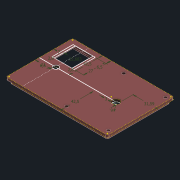
# Autodesk Inventor part: caja
Saved by Autodesk Inventor 2021 (Build 250183000, 183)
## iProperties
Created: 2021-12-14
Part Number: caja
Material: Generic
Document SubType Name: Modeling
Designer: Juan M. Casillas
Density: 1 g/cm^3
Appearance: Default
Author: Juan M. Casillas
Autodesk Inventor part; units mm, degrees
ref_plane "YZ Plane" through (0, 0, 0) normal (1, 0, 0) x (0, 1, 0)
ref_plane "XZ Plane" through (0, 0, 0) normal (0, 1, 0) x (-1, 0, 0)
ref_plane "XY Plane" through (0, 0, 0) normal (0, 0, 1) x (1, 0, 0)
sketch "Sketch1" plane through (0, 0, 0) normal (0, 1, 0) x (-1, 0, 0)
  line L0 (55, 45) -> (-55, 45)
  line L1 (-55, 45) -> (-55, -45)
  line L2 (-55, -45) -> (55, -45)
  line L3 (55, -45) -> (55, 45)
  line L4 (55, 45) -> (-55, -45) construction
  line L5 (-55, 45) -> (55, -45) construction
  line L6 (-12.1638, 34.5239) -> (-35.1638, 34.5239)
  line L7 (-35.1638, 34.5239) -> (-35.1638, 7.5239)
  line L8 (-35.1638, 7.5239) -> (-12.1638, 7.5239)
  line L9 (-12.1638, 7.5239) -> (-12.1638, 34.5239)
  line L10 (-12.1638, 34.5239) -> (-35.1638, 7.5239) construction
  line L11 (-35.1638, 34.5239) -> (-12.1638, 7.5239) construction
  circle A0 centre (-27.7205, -16.8019) radius 3.25
  line L12 (55, 0) -> (31, 0) construction
  circle A1 centre (31, 0) radius 4 construction
  circle A2 centre (31, 0) radius 40 construction
  point P0 (0, 0)
  point P1 (-23.6638, 21.0239)
  dimension "d1" = 110
  dimension "d2" = 90
  dimension "d3" = 23
  dimension "d4" = 27
  dimension "d5" = 6.5
  dimension "d6" = 24
  dimension "d7" = 8
  dimension "d8" = 80
  constraints: 26 end point, 5 midpoint, 4 parallel, 3 centre point, 3 horizontal, 2 coincident, 2 perpendicular
  measures "d1" distance of L2.end L1.end
  measures "d2" distance of L1.end L0.end
  measures "d3" distance of L8.end L7.end
  measures "d4" distance of L7.end L6.end
  measures "d5" diameter of A0
  measures "d6" distance of L12.start L12.end
  measures "d7" diameter of A1
  measures "d8" diameter of A2
sketch "Sketch2" plane through (0, 0, 0) normal (0, 1, 0) x (-1, 0, 0)
  line L0 (82.5, 45) -> (-40, 45)
  line L1 (-40, 45) -> (-40, -40)
  line L2 (-40, -40) -> (82.5, -40)
  line L3 (82.5, -40) -> (82.5, 45)
  line L4 (82.5, 45) -> (-40, -40) construction
  line L5 (-40, 45) -> (82.5, -40) construction
  point P0 (0, 0)
  dimension "d10" = 122.5
  dimension "d11" = 85
  constraints: 12 end point, 2 parallel, 1 horizontal, 1 perpendicular
  measures "d10" distance of L2.end L1.end
  measures "d11" distance of L1.end L0.end
extrude "Extrusion1" add sketch "Sketch2" along normal blind 3
sketch "Sketch3" plane through (0, 0, 0) normal (0, -1, 0) x (1, 0, 0)
  circle A0 centre (8.41, 2.5) radius 11.1
  circle A1 centre (8.41, 2.5) radius 14.1
  line L0 (40, 45) -> (40, -40) construction
  line L1 (-82.5, 45) -> (40, 45) construction
  line L2 (-82.5, -40) -> (-82.5, 45) construction
  line L3 (40, -40) -> (-82.5, -40) construction
  line L4 (40, 2.5) -> (-82.5, 2.5) construction
  circle A2 centre (8.41, 2.5) radius 4.5
  line L5 (-82.5, 2.5) -> (40, 2.5) construction
  dimension "d15" = 22.2
  dimension "d16" = 3
  dimension "d20" = 42.5
  dimension "d21" = 9
  dimension "d42" = 31.59
  constraints: 4 end point, 3 centre point, 2 coincident, 2 midpoint, 1 perpendicular, 1 point on line
  measures "d15" diameter of A0
  measures "d16" radial gap between concentric circles of A0 A1
  measures "d20" distance between parallel lines of L1 L4
  measures "d21" diameter of A2
  measures "d42" distance from line of L0 point (8.41, 2.5)
extrude "Extrusion2" add sketch "Sketch3" along normal blind 3.5 contours A1
thicken "Thicken1" operation add thickness 7 both sides no extend neighbours yes toward (-1, 0, 0) faces at (-82.5, 1, -11.6667)
fillet "Fillet1" radius 2 4 edges at (-89.5, 1.5, 45) (40, 1.5, 45) (40, 1.5, -40) (-89.5, 1.5, -40)
extrude "Extrusion3" cut sketch "Sketch3" against normal blind 10 contours A2
sketch "Sketch4" plane through (0, 0, 0) normal (0, -1, 0) x (1, 0, 0)
  arc A0 (-7.0479, 5.0014) -> (-5.1277, 6.4422) centre (-7.0479, 7.0014) ccw
  line L0 (-13.69, 5.0014) -> (-7.0479, 5.0014)
  arc A1 (-13.69, 5.0014) -> (-15.69, 3.0014) centre (-13.69, 3.0014) ccw
  line L1 (-15.69, 2.0014) -> (-15.69, 3.0014)
  arc A2 (-15.69, 2.0014) -> (-13.69, 0.0014) centre (-13.69, 2.0014) ccw
  line L2 (-7.0487, 0.0014) -> (-13.69, 0.0014)
  arc A3 (-5.1284, -1.4397) -> (-7.0487, 0.0014) centre (-7.0487, -1.9986) ccw
  arc A4 (-5.1277, 6.4422) -> (-5.1284, -1.4397) centre (8.41, 2.5) ccw
  circle A5 centre (8.41, 2.5) radius 14.1 projected
  line L3 (8.41, -14.9987) -> (8.41, 25.3428) construction
  arc A6 (21.9477, 6.4422) -> (23.8679, 5.0014) centre (23.8679, 7.0014) ccw
  line L4 (30.51, 5.0014) -> (23.8679, 5.0014)
  arc A7 (32.51, 3.0014) -> (30.51, 5.0014) centre (30.51, 3.0014) ccw
  arc A8 (21.9484, -1.4397) -> (21.9477, 6.4422) centre (8.41, 2.5) ccw
  arc A9 (23.8687, 0.0014) -> (21.9484, -1.4397) centre (23.8687, -1.9986) ccw
  line L5 (32.51, 2.0014) -> (32.51, 3.0014)
  arc A10 (30.51, 0.0014) -> (32.51, 2.0014) centre (30.51, 2.0014) ccw
  line L6 (23.8687, 0.0014) -> (30.51, 0.0014)
  point P0 (0, 0)
  point P1 (21.9477, 6.4422)
  point P2 (21.9484, -1.4397)
  constraints: 20 point on circle, 14 end point, 12 symmetric about line, 10 centre point, 1 concentric, 1 vertical, 5 other
extrude "Extrusion4" add sketch "Sketch4" along normal up to surface (3.5 mm away) contours A0 A4 A3 L2 A2 L1 A1 L0 | A6 L4 A7 L5 A10 L6 A9 A5
fillet "Fillet2" radius 2 16 edges at (27.189, 0, 5.0014) (31.9242, 0, 4.4156) (32.51, 0, 2.5014) (31.9242, 0, 0.5872) (27.1894, 0, 0.0014) (22.6683, 0, -0.3989) (8.41, 0, -11.6) (-5.8483, 0, -0.3989) (-10.3694, 0, 0.0014) (-15.1042, 0, 0.5872) (-15.69, 0, 2.5014) (-15.1042, 0, 4.4156) (-10.369, 0, 5.0014) (-5.8476, 0, 5.4017) (8.41, 0, 16.6) (22.6676, 0, 5.4017)
sketch "Sketch5" plane through (0, 0, 0) normal (0, -1, 0) x (1, 0, 0)
  arc A0 (-89.5, -38) -> (-87.5, -40) centre (-87.5, -38) ccw projected
  line L0 (38, -40) -> (-87.5, -40) projected
  arc A1 (38, -40) -> (40, -38) centre (38, -38) ccw projected
  line L1 (40, 43) -> (40, -38) projected
  arc A2 (40, 43) -> (38, 45) centre (38, 43) ccw projected
  line L2 (-87.5, 45) -> (38, 45) projected
  arc A3 (-87.5, 45) -> (-89.5, 43) centre (-87.5, 43) ccw projected
  line L3 (-89.5, -38) -> (-89.5, 43) projected
  line L4 (30.51, 7.0014) -> (23.8679, 7.0014) projected
  arc A4 (34.51, 3.0014) -> (30.51, 7.0014) centre (30.51, 3.0014) ccw projected
  line L5 (34.51, 2.0014) -> (34.51, 3.0014) projected
  arc A5 (30.51, -1.9986) -> (34.51, 2.0014) centre (30.51, 2.0014) ccw projected
  line L6 (23.8687, -1.9986) -> (30.51, -1.9986) projected
  arc A6 (-7.0487, -1.9986) -> (23.8687, -1.9986) centre (8.41, 2.5) ccw projected
  line L7 (-13.69, -1.9986) -> (-7.0487, -1.9986) projected
  arc A7 (-17.69, 2.0014) -> (-13.69, -1.9986) centre (-13.69, 2.0014) ccw projected
  line L8 (-17.69, 3.0014) -> (-17.69, 2.0014) projected
  arc A8 (-13.69, 7.0014) -> (-17.69, 3.0014) centre (-13.69, 3.0014) ccw projected
  line L9 (-7.0479, 7.0014) -> (-13.69, 7.0014) projected
  arc A9 (23.8679, 7.0014) -> (-7.0479, 7.0014) centre (8.41, 2.5) ccw projected
  line L10 (-84.9, 42.4) -> (35.4, 42.4)
  line L11 (37.4, 40.4) -> (37.4, -35.4)
  line L12 (35.4, -37.4) -> (-84.9, -37.4)
  line L13 (-86.9, -35.4) -> (-86.9, 40.4)
  arc A10 (-86.9, -35.4) -> (-84.9, -37.4) centre (-84.9, -35.4) ccw
  arc A11 (-84.9, 42.4) -> (-86.9, 40.4) centre (-84.9, 40.4) ccw
  arc A12 (37.4, 40.4) -> (35.4, 42.4) centre (35.4, 40.4) ccw
  arc A13 (35.4, -37.4) -> (37.4, -35.4) centre (35.4, -35.4) ccw
  line L14 (-84.9, -35.9) -> (35.4, -35.9)
  arc A14 (35.4, -35.9) -> (35.9, -35.4) centre (35.4, -35.4) ccw
  line L15 (35.9, -35.4) -> (35.9, 40.4)
  arc A15 (35.9, 40.4) -> (35.4, 40.9) centre (35.4, 40.4) ccw
  line L16 (35.4, 40.9) -> (-84.9, 40.9)
  arc A16 (-84.9, 40.9) -> (-85.4, 40.4) centre (-84.9, 40.4) ccw
  line L17 (-85.4, 40.4) -> (-85.4, -35.4)
  arc A17 (-85.4, -35.4) -> (-84.9, -35.9) centre (-84.9, -35.4) ccw
  point P0 (0, 0)
  dimension "d27" = 2.6
  dimension "d28" = 2
  dimension "d29" = 1.5
  constraints: 16 end point, 16 point on circle, 8 centre point, 8 tangent, 3 equal radius, 10 other
  measures "d27" distance between parallel lines of L3 L13
  measures "d28" radius of A10
  measures "d29" distance between parallel lines of L12 L14
extrude "Extrusion5" add sketch "Sketch5" along normal blind 4 contours L10 A12 L11 A13 L12 A10 L13 A11
fillet "Fillet3" radius 2 8 edges at (35.7536, 0, -35.7536) (35.9, 0, 2.5) (35.7536, 0, 40.7536) (-24.75, 0, 40.9) (-85.2536, 0, 40.7536) (-85.4, 0, 2.5) (-85.2536, 0, -35.7536) (-24.75, 0, -35.9)
sketch "Sketch6" plane through (0, -3.5, 0) normal (0, -1, 0) x (1, 0, 0)
  arc A0 (21.9477, 6.4422) -> (-5.1277, 6.4422) centre (8.41, 2.5) ccw construction
  arc A1 (-7.0479, 5.0014) -> (-5.1277, 6.4422) centre (-7.0479, 7.0014) ccw construction
  line L0 (-13.69, 5.0014) -> (-7.0479, 5.0014) construction
  arc A2 (-13.69, 5.0014) -> (-15.69, 3.0014) centre (-13.69, 3.0014) ccw construction
  line L1 (-15.69, 2.0014) -> (-15.69, 3.0014) construction
  arc A3 (-15.69, 2.0014) -> (-13.69, 0.0014) centre (-13.69, 2.0014) ccw construction
  line L2 (-7.0487, 0.0014) -> (-13.69, 0.0014) construction
  arc A4 (-5.1284, -1.4397) -> (-7.0487, 0.0014) centre (-7.0487, -1.9986) ccw construction
  arc A5 (-5.1284, -1.4397) -> (21.9484, -1.4397) centre (8.41, 2.5) ccw construction
  arc A6 (23.8687, 0.0014) -> (21.9484, -1.4397) centre (23.8687, -1.9986) ccw construction
  line L3 (30.51, 0.0014) -> (23.8687, 0.0014) construction
  arc A7 (30.51, 0.0014) -> (32.51, 2.0014) centre (30.51, 2.0014) ccw construction
  line L4 (32.51, 3.0014) -> (32.51, 2.0014) construction
  arc A8 (32.51, 3.0014) -> (30.51, 5.0014) centre (30.51, 3.0014) ccw construction
  line L5 (23.8679, 5.0014) -> (30.51, 5.0014) construction
  arc A9 (21.9477, 6.4422) -> (23.8679, 5.0014) centre (23.8679, 7.0014) ccw construction
  circle A10 centre (8.41, 2.5) radius 11.1 construction
  line L6 (-15.69, 2.5014) -> (32.51, 2.5014) construction
  line L7 (-15.69, 2.5014) -> (-10.69, 2.5014) construction
  point P0 (0, 0)
  point P1 (27.51, 2.5014)
  point P2 (27.51, 2.5014)
  dimension "d33" = 5
  dimension "d34" = 5
  constraints: 4 end point, 2 coincident, 2 midpoint, 2 point on line
  measures "d33" distance from line of L4 point (27.51, 2.501)
  measures "d34" distance of L6.start L7.end
hole "Hole1" at (-10.69, -3.5, 2.5014) at (27.51, -3.5, 2.5014) direction (0, 1, 0) diameter 3.42 depth 5
sketch "Sketch7" plane through (0, 3, 0) normal (0, 1, 0) x (1, 0, 0)
  circle A0 centre (8.41, -2.5) radius 4.5 construction
  arc A1 (-87.5, 40) -> (-89.5, 38) centre (-87.5, 38) ccw construction
  line L0 (-89.5, 38) -> (-89.5, -43) construction
  arc A2 (-89.5, -43) -> (-87.5, -45) centre (-87.5, -43) ccw construction
  line L1 (-87.5, -45) -> (38, -45) construction
  arc A3 (38, -45) -> (40, -43) centre (38, -43) ccw construction
  line L2 (40, -43) -> (40, 38) construction
  arc A4 (40, 38) -> (38, 40) centre (38, 38) ccw construction
  line L3 (38, 40) -> (-87.5, 40) construction
  line L4 (-68.5, 40) -> (-68.5, -45) construction
  line L5 (-40.8109, -2.5) -> (-89.5, -2.5) construction
  circle A5 centre (-68.5, -2.5) radius 3.3
  line L6 (-54.217, 33.5) -> (-82.5, 33.5)
  line L7 (-82.5, 33.5) -> (-82.5, 6.5)
  line L8 (-82.5, 6.5) -> (-54.217, 6.5)
  line L9 (-54.217, 6.5) -> (-54.217, 33.5)
  line L10 (-54.217, 33.5) -> (-57.017, 33.5)
  line L11 (-57.017, 33.5) -> (-57.017, 6.5)
  line L12 (-57.017, 6.5) -> (-54.217, 6.5)
  line L13 (-54.217, 6.5) -> (-54.217, 33.5)
  line L14 (-82.5, 33.5) -> (-79.7, 33.5)
  line L15 (-79.7, 33.5) -> (-79.7, 6.5)
  line L16 (-79.7, 6.5) -> (-82.5, 6.5)
  line L17 (-82.5, 6.5) -> (-82.5, 33.5)
  line L18 (8.41, -2.5) -> (-89.5, -2.5)
  point P0 (0, 0)
  dimension "d45" = 21
  dimension "d46" = 42.5
  dimension "d47" = 6.6
  dimension "d48" = 6.5
  dimension "d49" = 7
  dimension "d50" = 27
  dimension "d52" = 2.8
  dimension "d53" = 2.8
  dimension "d59" = 22.683
  constraints: 30 end point, 6 parallel, 5 perpendicular, 5 point on line, 3 horizontal, 3 midpoint, 1 centre point
  measures "d45" distance between parallel lines of L0 L4
  measures "d46" distance between parallel lines of L3 L5
  measures "d47" diameter of A5
  measures "d48" distance between parallel lines of L3 L6
  measures "d49" distance between parallel lines of L0 L7
  measures "d50" distance of L8.end L6.start
  measures "d52" distance of L12.end L11.end
  measures "d53" distance of L15.end L16.end
  measures "d59" distance between parallel lines of L11 L15
extrude "Extrusion6" cut sketch "Sketch7" against normal blind 4 contours L18 A5 | A5 L18 | L11 L8 L15 L6
sketch "Sketch8" plane through (0, 0, 0) normal (0, -1, 0) x (1, 0, 0)
  line L0 (-54.217, -6.5) -> (-54.217, -33.5) projected
  line L1 (-57.017, -6.5) -> (-54.217, -6.5) projected
  line L2 (-57.017, -33.5) -> (-57.017, -6.5) projected
  line L3 (-54.217, -33.5) -> (-57.017, -33.5) projected
  line L4 (-82.5, -33.5) -> (-79.7, -33.5) projected
  line L5 (-82.5, -6.5) -> (-82.5, -33.5) projected
  line L6 (-82.5, -6.5) -> (-54.217, -6.5) projected
  line L7 (-79.7, -6.5) -> (-79.7, -33.5) projected
  point P0 (0, 0)
extrude "Extrusion7" cut sketch "Sketch8" against normal blind 1.2
thicken "Thicken2" operation add thickness 0.2 both sides no extend neighbours yes toward (0, 0, 1) faces at (-72.139, 2.4, -6.5) (-57.017, 2.4, -15.5) (-64.578, 1.8, -33.5) (-79.7, 2.4, -24.5)
sketch "Sketch9" plane through (0, 3, 0) normal (0, 1, 0) x (1, 0, 0)
  circle A0 centre (8.41, -2.5) radius 40 construction
  line L0 (38, 38) -> (8.41, -2.5) construction
  line L1 (8.41, -2.5) -> (38, -43) construction
  line L2 (38, 38) -> (35.0503, 33.9628) construction
  line L3 (38, -43) -> (35.0503, -38.9628) construction
  line L4 (30.7963, -33.1402) -> (-23.0057, 40.4988) construction
  line L5 (21.8569, 15.9049) -> (-24.0625, -46.9453) construction
  line L6 (35.0503, 33.9628) -> (-18.2303, 33.9628)
  line L7 (-18.2303, 33.9628) -> (-18.2303, -38.9628)
  line L8 (-18.2303, -38.9628) -> (35.0503, -38.9628)
  line L9 (35.0503, -38.9628) -> (35.0503, 33.9628)
  point P0 (0, 0)
  dimension "d64" = 80
  dimension "d65" = 5
  dimension "d66" = 5
  constraints: 20 end point, 7 point on line, 5 coincident, 2 parallel, 1 centre point, 1 horizontal, 1 perpendicular
  measures "d64" diameter of A0
  measures "d65" distance of L2.start L2.end
  measures "d66" distance of L1.end L3.end
hole "Hole2" at (35.0503, 3, -33.9628) at (35.0503, 3, 38.9628) at (-18.2303, 3, -33.9628) at (-18.2303, 3, 38.9628) direction (0, -1, 0) diameter 4 depth 2.5
body "Solid1"
